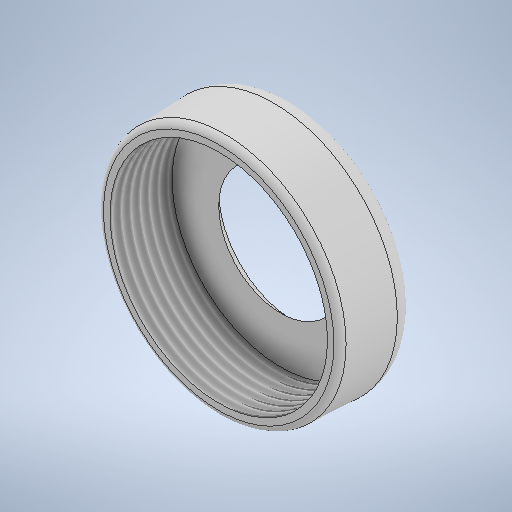
# Autodesk Inventor part: Deckel
Saved by Autodesk Inventor 2025.1 (Build 291241000, 241)
## iProperties
Created: 2025-01-26
Part Number: Deckel
Material: Generisch
Document SubType Name: Modeling
Designer: joebe
Density: 1 g/cm^3
Appearance: Vorgabe
Author: joebe
Autodesk Inventor part; units mm, degrees
ref_plane "YZ Plane" through (0, 0, 0) normal (1, 0, 0) x (0, 1, 0)
ref_plane "XZ Plane" through (0, 0, 0) normal (0, 1, 0) x (-1, 0, 0)
ref_plane "XY Plane" through (0, 0, 0) normal (0, 0, 1) x (1, 0, 0)
sketch "Skizze1" plane through (0, 0, 0) normal (0, 0, 1) x (1, 0, 0)
  line L0 (10, 12) -> (20, 12)
  line L1 (20, 12) -> (19.5, 0)
  line L2 (19.5, 0) -> (17.5, 0)
  line L3 (17.5, 0) -> (17.5, 10)
  line L4 (17.5, 10) -> (10, 10)
  line L5 (10, 10) -> (10, 12)
  line L6 (0, 0) -> (0, 8.6013)
  line L7 (18.5, 0) -> (18.5, 1.5)
  line L8 (18.5, 1.5) -> (17.5, 1.5)
  dimension "d0" = 35
  dimension "d1" = 10
  dimension "d2" = 20
  dimension "d4" = 2
  dimension "d9" = 10
  dimension "d10" = 2
  dimension "d15" = 1
  dimension "d16" = 1.5
  constraints: 18 end point, 4 perpendicular, 2 vertical, 1 horizontal, 1 horizontal alignment, 1 midpoint, 1 point on line
  measures "d0" diameter of L3 L6
  measures "d1" distance of L2.end L3.end
  measures "d2" diameter of L5 L6
  measures "d4" distance between parallel lines of L0 L4
  measures "d9" distance of L0.start L0.end
  measures "d10" distance of L1.end L2.end
  measures "d15" distance of L7.end L8.end
  measures "d16" distance of L7.start L7.end
revolve "Umdrehung1" add sketch "Skizze1" angle 360 about axis through (0, 0, 0) along (0, 1, 0)
chamfer "Fasen1" distance 2 angle 45 1 edges at (-10, 12, 0)
thread "Gewinde1" size "M35x1.5" class "6H" standard "ISO Metric profile" full length
fillet "Rundung1" radius 3 1 edges at (-20, 12, 0)
fillet "Rundung2" radius 1 1 edges at (-19.5, 0, 0)
